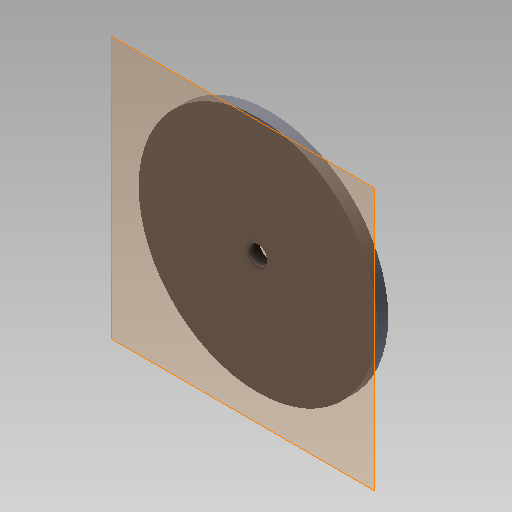
# Autodesk Inventor part: PWTR-0038
Saved by Autodesk Inventor 2020 (Build 240168000, 168)
## iProperties
Part Number: PWTR-0038
Document SubType Name: Modeling
Created: 2003-02-05
Designer: B. BOGAN
Material: Stainless Steel, 303
Description: TROWEL PITCH PLATE
Mass: 297.38 g
Surface Area: 177.539 cm^2
Volume: 38.3717 cm^3
Density: 7.75 g/cm^3
Appearance: Steel
Vendor: Non-Design Specific
Control State: 0
Master: False
Checked Out: False
Shininess: 64.0
Length Units: 11272
Angle Units: 11279
Time Units: 11290
Mass Units: 11286
Length Display Precision: 3
Angle Display Precision: 2
Compacted: True
Density: 0.0
Volumn: 0.0
Area: 0.0
PropertySet Name: Model Information
Title: PITCH PLATE
Author: B. BOGAN
Revision Number: B
Autodesk Inventor part; units mm, degrees
ref_plane "YZ Plane" through (0, 0, 0) normal (1, 0, 0) x (0, 1, 0)
ref_plane "XZ Plane" through (0, 0, 0) normal (0, 1, 0) x (-1, 0, 0)
ref_plane "XY Plane" through (0, 0, 0) normal (0, 0, 1) x (1, 0, 0)
sketch "Sketch1" plane through (0, 0, 0) normal (0, 0, 1) x (1, 0, 0)
  circle A0 centre (0, 0) radius 50.8
  dimension "d0" = 101.6
  constraints: 1 centre point
  measures "d0" diameter of A0
extrude "Extrusion1" add sketch "Sketch1" along normal blind 4.7625
sketch "Sketch2" plane through (0, 0, 4.7625) normal (0, 0, 1) x (1, 0, 0)
  circle A0 centre (0, 0) radius 50.8 projected
hole "Hole1" at (0, 0, 4.7625) direction (0, 0, -1) diameter 8.001 end through all
ref_plane "Work Plane1" through (0, 0, 11.1125) normal (0, 0, 1) x (1, 0, 0)
body "Solid1"
